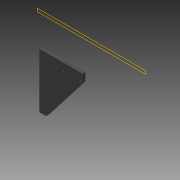
# Autodesk Inventor part: side support
Saved by Autodesk Inventor 2014 (Build 180170000, 170)
## iProperties
Created: 2013-07-28
Part Number: side support
Material: Generic
Document SubType Name: Modeling
Designer: employee
Density: 1 g/cm^3
Mass: 395.994 g
Surface Area: 741.582 cm^2
Volume: 395.994 cm^3
Appearance: Gray
d2: 9.843 in
d3: 0.502 in
d4: 0.00 deg
d5: 0.787 in
d6: 1.083 in
d8: 0.00 deg
d9: 0.134 in
d11: 0.256 in
d12: 0.118 in
Author: employee
Autodesk Inventor part; units mm, degrees
ref_plane "YZ Plane" through (0, 0, 0) normal (1, 0, 0) x (0, 1, 0)
ref_plane "XZ Plane" through (0, 0, 0) normal (0, 1, 0) x (-1, 0, 0)
ref_plane "XY Plane" through (0, 0, 0) normal (0, 0, 1) x (1, 0, 0)
ref_plane "Work Plane1" through (0, 142.0555, 0) normal (0, 0, 1) x (1, 0, 0)
sketch "Sketch1" plane through (0, 142.0555, 0) normal (0, 0, 1) x (1, 0, 0)
  line L0 (450, -129.5555) -> (450, -142.0555) projected
  line L1 (0, -129.5555) -> (450, -129.5555) projected
  line L2 (0, -142.0555) -> (0, -129.5555) projected
  line L3 (450, -142.0555) -> (0, -142.0555) projected
  circle A0 centre (109.7339, -163.0555) radius 4.05 projected
  circle A1 centre (184.7339, -163.0555) radius 4.05 projected
  line L4 (92.2339, -147.0555) -> (92.2339, -142.0555) projected
  arc A2 (97.2339, -152.0555) -> (92.2339, -147.0555) centre (92.2339, -152.0555) ccw projected
  line L5 (97.2339, -152.0555) -> (97.2339, -163.0555) projected
  arc A3 (97.2339, -163.0555) -> (122.2339, -163.0555) centre (109.7339, -163.0555) ccw projected
  line L6 (122.2339, -163.0555) -> (122.2339, -152.0555) projected
  arc A4 (127.2339, -147.0555) -> (122.2339, -152.0555) centre (127.2339, -152.0555) ccw projected
  line L7 (127.2339, -147.0555) -> (167.2339, -147.0555) projected
  arc A5 (172.2339, -152.0555) -> (167.2339, -147.0555) centre (167.2339, -152.0555) ccw projected
  line L8 (172.2339, -152.0555) -> (172.2339, -163.0555) projected
  arc A6 (172.2339, -163.0555) -> (197.2339, -163.0555) centre (184.7339, -163.0555) ccw projected
  line L9 (197.2339, -163.0555) -> (197.2339, -152.0555) projected
  arc A7 (202.2339, -147.0555) -> (197.2339, -152.0555) centre (202.2339, -152.0555) ccw projected
  line L10 (202.2339, -142.0555) -> (202.2339, -147.0555) projected
  line L11 (92.2339, -142.0555) -> (202.2339, -142.0555) projected
  line L12 (0, -129.5555) -> (0, -379.5555)
  line L13 (0, -379.5555) -> (27.5, -379.5555)
  line L14 (35.3974, -375.6899) -> (194.6057, -170.7235)
  line L15 (197.2339, -163.0555) -> (197.2339, -129.5555)
  line L16 (0, -129.5555) -> (197.2339, -129.5555)
  arc A8 (194.6057, -170.7235) -> (197.2339, -163.0555) centre (184.7339, -163.0555) ccw
  arc A9 (27.5, -379.5555) -> (35.3974, -375.6899) centre (27.5, -369.5555) ccw
  dimension "d2" = 250
  dimension "d5" = 20
  dimension "d6" = 27.5
  constraints: 10 end point, 5 point on circle, 5 tangent, 4 perpendicular, 2 centre point, 1 point on line
  measures "d2" distance of L1.start L12.end
  measures "d5" diameter of A9
  measures "d6" distance from line of A9.centre L12
extrude "Extrusion1" add sketch "Sketch1" along normal blind 12.7508 contours L15 L3 L2 L1 | L15 L9 A6 L8 A5 L7 A4 L6 A3 L5 A2 L4 L3 | L3 L4 A2 L5 A3 L6 A4 L7 A5 L8 A6 L14 A9 L13 L12
sketch "Sketch2" plane through (0, 142.0555, 0) normal (0, 0, -1) x (-1, 0, 0)
  circle A0 centre (-27.5, -369.5555) radius 1.55
  circle A1 centre (-27.5, -157.0555) radius 1.55
  point P0 (0, -142.0555)
  constraints: 2 centre point, 4 other
extrude "Extrusion2" cut sketch "Sketch2" against normal through all
sketch "Sketch3" plane through (0, 142.0555, 12.7508) normal (0, 0, 1) x (1, 0, 0)
  circle A0 centre (27.5, -157.0555) radius 1.55 projected
  arc A1 (27.5, -379.5555) -> (35.3974, -375.6899) centre (27.5, -369.5555) ccw projected
  point P0 (0, -142.0555)
hole "Hole1" at (27.5, -15, 12.7508) at (27.5, -227.5, 12.7508) direction (0, 0, -1) diameter 3.4036 end through all counterbore diameter 6.5024 counterbore depth 2.9972 clearance for "Socket Head Cap Screw" size "M3" standard "Ansi Metric M Profile"
body "Solid1"
